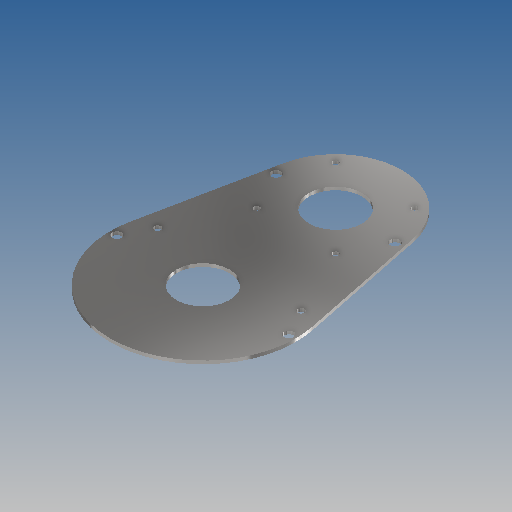
# Autodesk Inventor part: PWTR-0128
Saved by Autodesk Inventor 2021.1 (Build 251245000, 245)
## iProperties
Created: 2020-08-28
Part Number: PWTR-0128
Material: Aluminum 6061
Document SubType Name: Modeling
Designer: alid
Density: 2.7 g/cm^3
Appearance: Steel - Polished
Description: Drive Unit Backing Plate
Author: alid
Revision Number: A
Autodesk Inventor part; units mm, degrees
ref_plane "YZ Plane" through (0, 0, 0) normal (1, 0, 0) x (0, 1, 0)
ref_plane "XZ Plane" through (0, 0, 0) normal (0, 1, 0) x (-1, 0, 0)
ref_plane "XY Plane" through (0, 0, 0) normal (0, 0, 1) x (1, 0, 0)
sketch "Sketch1" plane through (0, 0, 0) normal (0, 0, 1) x (1, 0, 0)
  circle A0 centre (0, 0) radius 52.5 construction
  circle A1 centre (0, 0) radius 25
  circle A2 centre (0, 0) radius 62.5
  line L0 (0, 0) -> (0, 52.5) construction
  line L1 (0, 0) -> (37.1231, 37.1231) construction
  line L2 (0, 0) -> (0, -125) construction
  circle A3 centre (0, -125) radius 87.5
  line L3 (-85.7321, -107.5) -> (-61.2372, 12.5)
  line L4 (85.7321, -107.5) -> (61.2372, 12.5)
  circle A4 centre (0, -125) radius 25
  circle A5 centre (0, -125) radius 81 construction
  circle A6 centre (0, 0) radius 56 construction
  line L5 (0, 0) -> (-56, 0) construction
  line L6 (0, -125) -> (-81, -125) construction
  dimension "d31" = 162
  dimension "d32" = 112
  dimension "d0" = 105
  dimension "d1" = 50
  dimension "d2" = 125
  dimension "d3" = 45
  dimension "d4" = 125
  dimension "d5" = 175
  dimension "d6" = 50
  constraints: 14 end point, 7 coincident, 6 point on circle, 5 centre point, 4 tangent, 2 horizontal alignment, 2 vertical, 1 horizontal, 1 parallel, 4 other
  measures "d0" diameter of A0
  measures "d1" diameter of A1
  measures "d2" diameter of A2
  measures "d3" angle of L0 L1
  measures "d4" distance of L0.start L2.end
  measures "d5" diameter of A3
  measures "d6" diameter of A4
extrude "Extrusion1" add sketch "Sketch1" along normal blind 3
sketch "Sketch2" plane through (0, 0, 0) normal (0, 0, 1) x (1, 0, 0)
  line L0 (0, 0) -> (0, -100)
  line L1 (67.5, -100) -> (-67.5, -100)
  arc A0 (-85.7321, -107.5) -> (85.7321, -107.5) centre (0, -125) ccw projected
  dimension "d11" = 100
  dimension "d12" = 135
  dimension "d40" = 25
  constraints: 4 end point, 1 horizontal, 1 midpoint, 1 vertical
  measures "d11" distance of L0.end L0.start
  measures "d12" distance of L1.start L1.end
  measures "d40" distance from line of A0.centre L1
hole "Hole1" at (67.5, -100, 0) at (-67.5, -100, 0) direction (0, 0, 1) diameter 6.6 end through all clearance for "Hex Head Cap Screw ISO 24017" size "M6" standard "ISO"
hole "Hole2" at (37.1231, 37.1231, 0) direction (0, 0, 1) diameter 5.5 end through all clearance for "Hex Head Cap Screw ISO 24017" size "M5" standard "ISO"
pattern_circular "Circular Pattern1" count 4 over 360 about axis through (0, 0, 0) along (0, 0, 1) of "Hole2"
hole "Hole3" at (-56, 0, 0) at (-81, -125, 0) direction (0, 0, 1) diameter 9 end through all
mirror "Mirror1" about plane through (0, 0, 0) normal (1, 0, 0) of "Hole3"
body "Solid1"
